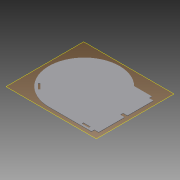
# Autodesk Inventor part: Foam_Right
Saved by Autodesk Inventor 2014 SP1 (Build 180222100, 222)
## iProperties
Created: 2014-02-22
Part Number: Foam_Right
Material: Generic
Document SubType Name: Modeling
Designer: tuleu
Density: 1 g/cm^3
Appearance: Default
Author: tuleu
Autodesk Inventor part; units mm, degrees
ref_plane "YZ Plane" through (0, 0, 0) normal (1, 0, 0) x (0, 1, 0)
ref_plane "XZ Plane" through (0, 0, 0) normal (0, 1, 0) x (-1, 0, 0)
ref_plane "XY Plane" through (0, 0, 0) normal (0, 0, 1) x (1, 0, 0)
ref_plane "Work Plane1" through (0, 0, 0) normal (0, 0, 1) x (1, 0, 0)
sketch "Sketch1" plane through (0, 0, 0) normal (0, 0, 1) x (1, 0, 0)
  arc A0 (157.2336, 394.4305) -> (-185.695, -445.5695) centre (-185.695, 44.4305) ccw construction
  line L0 (404.305, 394.4305) -> (404.305, 354.4305) construction
  line L1 (404.305, 354.4305) -> (524.305, 354.4305) construction
  line L2 (524.305, -5.5695) -> (404.305, -5.5695) construction
  line L3 (404.305, -5.5695) -> (404.305, -45.5695) construction
  line L4 (404.305, -45.5695) -> (524.305, -45.5695) construction
  line L5 (404.305, -405.5695) -> (404.305, -445.5695) construction
  line L6 (524.305, -405.5695) -> (404.305, -405.5695) construction
  line L7 (-185.695, -445.5695) -> (464.305, -445.5695) construction
  line L8 (404.305, 394.4305) -> (404.305, 354.4305)
  line L9 (464.305, 354.4305) -> (404.305, 354.4305)
  line L10 (404.305, -5.5695) -> (464.305, -5.5695)
  line L11 (404.305, -5.5695) -> (404.305, -45.5695)
  line L12 (464.305, -45.5695) -> (404.305, -45.5695)
  line L13 (404.305, -405.5695) -> (464.305, -405.5695)
  line L14 (404.305, -405.5695) -> (404.305, -445.5695)
  line L15 (464.305, 354.4305) -> (464.305, -5.5695)
  line L16 (464.305, -45.5695) -> (464.305, -405.5695)
  line L17 (404.305, -445.5695) -> (-185.695, -445.5695)
  line L18 (157.2336, 394.4305) -> (404.305, 394.4305)
  arc A1 (157.2336, 394.4305) -> (-185.695, -445.5695) centre (-185.695, 44.4305) ccw
  arc A2 (-521.5707, -227.8057) -> (-528.6418, -227.8057) centre (-525.1062, -231.3412) ccw projected
  line L19 (-539.2484, -238.4123) -> (-528.6418, -227.8057) projected
  arc A3 (-539.2484, -238.4123) -> (-539.2484, -245.4833) centre (-535.7128, -241.9478) ccw projected
  line L20 (-475.6088, -309.1229) -> (-539.2484, -245.4833) projected
  line L21 (-521.5707, -227.8057) -> (-457.9311, -291.4453) projected
  arc A4 (-457.9311, -298.5163) -> (-457.9311, -291.4453) centre (-461.4666, -294.9808) ccw projected
  arc A5 (-475.6088, -309.1229) -> (-468.5377, -309.1229) centre (-472.0732, -305.5874) ccw projected
  line L22 (-457.9311, -298.5163) -> (-468.5377, -309.1229) projected
  line L23 (249.305, -395.5695) -> (339.305, -395.5695) projected
  arc A6 (344.305, -400.5695) -> (339.305, -395.5695) centre (339.305, -400.5695) ccw projected
  line L24 (344.305, -400.5695) -> (344.305, -415.5695) projected
  arc A7 (339.305, -420.5695) -> (344.305, -415.5695) centre (339.305, -415.5695) ccw projected
  line L25 (339.305, -420.5695) -> (249.305, -420.5695) projected
  arc A8 (244.305, -415.5695) -> (249.305, -420.5695) centre (249.305, -415.5695) ccw projected
  line L26 (244.305, -415.5695) -> (244.305, -400.5695) projected
  arc A9 (249.305, -395.5695) -> (244.305, -400.5695) centre (249.305, -400.5695) ccw projected
  point P0 (0, 0)
  constraints: 23 end point, 4 collinear, 4 midpoint, 3 perpendicular, 2 parallel, 2 point on circle, 1 centre point, 1 coincident, 1 tangent
extrude "Extrusion1" add sketch "Sketch1" along normal blind 7
body "Solid1"
